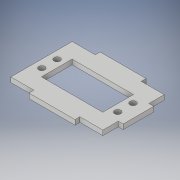
# Autodesk Inventor part: HOMBRO_SOST.SERVO
Saved by Autodesk Inventor 2019 (Build 230136000, 136)
## iProperties
Created: 2020-02-12
Part Number: HOMBRO_SOST.SERVO
Material: Genérico
Document SubType Name: Modeling
Designer: omar-
Density: 1 g/cm^3
Appearance: Valor por defecto
Author: omar-
Autodesk Inventor part; units mm, degrees
ref_plane "YZ Plane" through (0, 0, 0) normal (1, 0, 0) x (0, 1, 0)
ref_plane "XZ Plane" through (0, 0, 0) normal (0, 1, 0) x (-1, 0, 0)
ref_plane "XY Plane" through (0, 0, 0) normal (0, 0, 1) x (1, 0, 0)
sketch "Boceto1" plane through (0, 0, 0) normal (0, 1, 0) x (-1, 0, 0)
  circle A0 centre (0, 0) radius 5
  line L0 (10.1, 10) -> (-29.9, 10)
  line L1 (-29.9, 10) -> (-29.9, -10)
  line L2 (-29.9, -10) -> (10.1, -10)
  line L3 (10.1, -10) -> (10.1, 10)
  circle A1 centre (-34.66, 5) radius 2
  circle A2 centre (14.85, -5) radius 2
  circle A3 centre (14.85, 5) radius 2
  circle A4 centre (-34.66, -5) radius 2
  line L4 (20, 20) -> (-40, 20)
  line L5 (-40, 20) -> (-40, -20)
  line L6 (-40, -20) -> (20, -20)
  line L7 (20, -20) -> (20, 20)
  line L8 (5, 23.18) -> (-25, 23.18)
  line L9 (-25, 23.18) -> (-25, 20)
  line L10 (-25, 20) -> (5, 20)
  line L11 (5, 20) -> (5, 23.18)
  line L12 (5, -20) -> (-25, -20)
  line L13 (-25, -20) -> (-25, -23.18)
  line L14 (-25, -23.18) -> (5, -23.18)
  line L15 (5, -23.18) -> (5, -20)
  line L16 (-40, 10) -> (-43.18, 10)
  line L17 (-43.18, 10) -> (-43.18, -10)
  line L18 (-43.18, -10) -> (-40, -10)
  line L19 (-40, -10) -> (-40, 10)
  dimension "d0" = 10
  dimension "d1" = 10
  dimension "d2" = 20
  dimension "d3" = 10.1
  dimension "d4" = 40
  dimension "d5" = 4
  dimension "d6" = 4
  dimension "d7" = 4
  dimension "d8" = 5
  dimension "d9" = 10
  dimension "d10" = 14.85
  dimension "d11" = 14.85
  dimension "d12" = 4
  dimension "d13" = 34.66
  dimension "d14" = 34.66
  dimension "d15" = 5
  dimension "d16" = 10
  dimension "d25" = 40
  dimension "d26" = 60
  dimension "d27" = 20
  dimension "d28" = 20
  dimension "d29" = 3.18
  dimension "d30" = 30
  dimension "d31" = 15
  dimension "d32" = 20
  dimension "d33" = 10
  dimension "d34" = 3.18
  constraints: 40 end point, 10 parallel, 5 centre point, 5 horizontal, 5 perpendicular, 4 collinear, 3 coincident, 2 equal length
  measures "d0" diameter of A0
  measures "d1" distance from line of L2 point (0, 0)
  measures "d2" distance of L2.end L0.start
  measures "d3" distance from line of point (0, 0) L3
  measures "d4" distance of L1.end L2.end
  measures "d5" diameter of A1
  measures "d6" diameter of A2
  measures "d7" diameter of A3
  measures "d8" vertical distance of point (0, 0) A3.centre
  measures "d9" distance of A2.centre A3.centre
  measures "d10" horizontal distance of point (0, 0) A3.centre
  measures "d11" horizontal distance of point (0, 0) A2.centre
  measures "d12" diameter of A4
  measures "d13" horizontal distance of A4.centre point (0, 0)
  measures "d14" horizontal distance of A1.centre point (0, 0)
  measures "d15" vertical distance of A4.centre point (0, 0)
  measures "d16" distance of A4.centre A1.centre
  measures "d25" distance of L6.end L4.start
  measures "d26" distance of L5.end L6.end
  measures "d27" distance from line of L6 point (0, 0)
  measures "d28" distance from line of L7 point (0, 0)
  measures "d29" distance of L14.end L12.start
  measures "d30" distance of L13.end L14.end
  measures "d31" distance between parallel lines of L15 L7
  measures "d32" distance of L16.end L17.end
  measures "d33" distance between parallel lines of L16 L4
  measures "d34" distance of L17.end L18.end
extrude "Extrusión1" add sketch "Boceto1" along normal blind 3.18 contours L7 L6 L5 L4 | L4 L9 L8 L11 | L15 L14 L13 L6 | L5 L18 L17 L16
